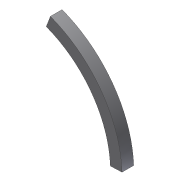
# Autodesk Inventor part: Frame_BottomGuideRail
Saved by Autodesk Inventor 2012 (Build 160160000, 160)
## iProperties
Created: 2012-01-11
Part Number: Frame_BottomGuideRail
Material: Default
Document SubType Name: Modeling
Designer: JesseK
Density: 1 g/cm^3
Author: JesseK
Autodesk Inventor part; units mm, degrees
ref_plane "YZ Plane" through (0, 0, 0) normal (1, 0, 0) x (0, 1, 0)
ref_plane "XZ Plane" through (0, 0, 0) normal (0, 1, 0) x (-1, 0, 0)
ref_plane "XY Plane" through (0, 0, 0) normal (0, 0, 1) x (1, 0, 0)
sketch "Sketch1" plane through (0, 0, 0) normal (0, 0, 1) x (1, 0, 0)
  arc A0 (241.112, 10.0687) -> (56.7808, 234.547) centre (0, 0) ccw
  arc A1 (215.712, 9.008) -> (50.7992, 209.8386) centre (0, 0) ccw
  line L0 (241.112, 10.0687) -> (215.712, 9.008)
  line L1 (56.7808, 234.547) -> (50.7992, 209.8386)
  line L2 (56.7808, 234.547) -> (0, 0) construction
  line L3 (0, 0) -> (241.112, 10.0687) construction
  point P0 (0, 0)
  dimension "d0" = 74
  dimension "d1" = 25.4
  dimension "d2" = 215.9
  constraints: 8 end point, 5 point on circle, 2 centre point, 2 coincident, 2 collinear
  measures "d0" angle of L0 L1
  measures "d1" horizontal distance of L0.start L0.end
  measures "d2" radius of A1
extrude "Extrusion1" add sketch "Sketch1" along normal blind 25.4
shell "Shell1" thickness 1.5875 removed faces 2 at (232.6453, 9.7152, 8.4667) at (52.7931, 218.0748, 8.4667)
sketch "Sketch2" plane through (0, 0, 25.4) normal (0, 0, 1) x (1, 0, 0)
  line L0 (50.7992, 209.8386) -> (56.7808, 234.547) projected
  arc A0 (215.712, 9.008) -> (50.7992, 209.8386) centre (0, 0) ccw projected
  line L1 (56.7808, 234.547) -> (50.7992, 209.8386)
  arc A1 (76.1992, 202.0062) -> (50.7992, 209.8386) centre (0, 0) ccw
  arc A2 (85.1716, 225.7923) -> (56.7808, 234.547) centre (0, 0) ccw
  line L2 (76.1992, 202.0062) -> (85.1716, 225.7923)
  line L3 (0, 0) -> (76.1992, 202.0062) construction
  line L4 (50.7992, 209.8386) -> (76.1992, 202.0062) construction
  dimension "d6" = 25.4
  constraints: 8 end point, 4 point on circle, 2 centre point, 2 coincident, 2 collinear
  measures "d6" horizontal distance of L0.start L2.start
extrude "Extrusion2" cut sketch "Sketch2" against normal through all
body "Solid1"
